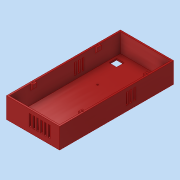
# Autodesk Inventor part: power_supply_case
Saved by Autodesk Inventor 2022 (Build 260153000, 153)
## iProperties
Created: 2020-11-03
Part Number: power_supply_case
Material: Generic
Document SubType Name: Modeling
Designer: nnico
Density: 1 g/cm^3
Appearance: Red
Author: nnico
Autodesk Inventor part; units mm, degrees
ref_plane "YZ Plane" through (0, 0, 0) normal (1, 0, 0) x (0, 1, 0)
ref_plane "XZ Plane" through (0, 0, 0) normal (0, 1, 0) x (-1, 0, 0)
ref_plane "XY Plane" through (0, 0, 0) normal (0, 0, 1) x (1, 0, 0)
sketch "Sketch1" plane through (0, 0, 0) normal (0, 1, 0) x (-1, 0, 0)
  line L0 (70, -150) -> (-70, -150)
  line L1 (-70, -150) -> (-70, 150)
  line L2 (-70, 150) -> (70, 150)
  line L3 (70, 150) -> (70, -150)
  line L4 (0, -150) -> (0, 150) construction
  line L5 (70, 0) -> (-70, 0) construction
  point P0 (0, 0)
  point P1 (0, 0)
  dimension "d0" = 140
  dimension "d1" = 300
  constraints: 12 end point, 5 midpoint, 2 parallel, 1 coincident, 1 horizontal, 1 perpendicular
  measures "d0" distance of L1.end L2.end
  measures "d1" distance of L0.end L1.end
extrude "Extrusion1" add sketch "Sketch1" along normal blind 4
sketch "Sketch2" plane through (0, 4, 0) normal (0, 1, 0) x (1, 0, 0)
  line L0 (-70, -150) -> (70, -150) projected
  line L1 (70, -150) -> (70, 150) projected
  line L2 (-70, -150) -> (70, -150)
  line L3 (70, -150) -> (70, 150)
  line L4 (70, 150) -> (-70, 150)
  line L5 (-70, 150) -> (-70, -150)
  line L6 (-66, -146) -> (66, -146)
  line L7 (66, -146) -> (66, 146)
  line L8 (66, 146) -> (-66, 146)
  line L9 (-66, 146) -> (-66, -146)
  point P0 (0, 0)
  dimension "d4" = 4
  dimension "d5" = 4
  dimension "d6" = 4
  dimension "d7" = 4
  constraints: 16 end point, 4 parallel, 2 horizontal, 2 perpendicular
  measures "d4" distance between parallel lines of L5 L9
  measures "d5" distance between parallel lines of L1 L7
  measures "d6" distance between parallel lines of L6 L0
  measures "d7" distance between parallel lines of L4 L8
extrude "Extrusion2" add sketch "Sketch2" along normal blind 50
sketch "Sketch3" plane through (0, 54, 0) normal (0, 1, 0) x (1, 0, 0)
  line L0 (-70, 150) -> (-70, -150) projected
  line L1 (-70, -90) -> (-60, -90)
  line L2 (-60, -90) -> (-60, -80)
  line L3 (-60, -80) -> (-70, -80)
  line L4 (-70, -80) -> (-70, -90)
  line L5 (-70, -150) -> (70, -150) projected
  line L6 (0, -150) -> (0, 150) construction
  line L7 (-70, 150) -> (70, 150) construction
  line L8 (70, -150) -> (70, 150) construction
  line L9 (70, 0) -> (-70, 0) construction
  line L10 (-70, 90) -> (-60, 90)
  line L11 (-60, 90) -> (-60, 80)
  line L12 (-60, 80) -> (-70, 80)
  line L13 (-70, 80) -> (-70, 90)
  line L14 (70, -90) -> (60, -90)
  line L15 (60, -90) -> (60, -80)
  line L16 (60, -80) -> (70, -80)
  line L17 (70, -80) -> (70, -90)
  line L18 (60, 90) -> (60, 80)
  line L19 (70, 90) -> (60, 90)
  line L20 (70, 80) -> (70, 90)
  line L21 (60, 80) -> (70, 80)
  line L22 (65, 80) -> (65, 90) construction
  line L23 (60, 85) -> (70, 85) construction
  circle A0 centre (65, 85) radius 2.5
  circle A1 centre (-65, 85) radius 2.5
  circle A2 centre (65, -85) radius 2.5
  circle A3 centre (-65, -85) radius 2.5
  point P0 (0, 0)
  dimension "d10" = 10
  dimension "d11" = 10
  dimension "d12" = 60
  dimension "d15" = 5
  constraints: 40 end point, 15 symmetric about line, 9 midpoint, 4 centre point, 2 parallel, 1 horizontal, 1 perpendicular, 1 point on line, 3 other
  measures "d10" distance of L3.end L2.end
  measures "d11" distance of L2.end L1.end
  measures "d12" distance from line of L5 L1.start
  measures "d15" diameter of A0
extrude "Extrusion3" add sketch "Sketch3" against normal blind 16 contours L10 L11 L12 L0 | L3 L2 L1 L0 | L14 L15 L16 L17 | L19 L20 L21 L18 | A0 | A1 | A2 | A3
sketch "Sketch4" plane through (0, 54, 0) normal (0, 1, 0) x (1, 0, 0)
  line L0 (70, -150) -> (-70, -150) construction
  line L1 (0, -150) -> (0, 150) construction
  line L2 (-70, 150) -> (70, 150) construction
  line L3 (70, -150) -> (70, 150) construction
  line L4 (70, 0) -> (-70, 0) construction
  line L5 (-70, -150) -> (-70, 150) construction
  line L6 (60, 90) -> (66, 90) construction
  line L7 (60, 90) -> (70, 90) construction
  line L8 (70, 90) -> (70, 80) construction
  line L9 (70, 80) -> (60, 80) construction
  line L10 (60, 80) -> (60, 90) construction
  line L11 (66, 80) -> (60, 80) construction
  line L12 (65, 90) -> (65, 80) construction
  line L13 (60, 80) -> (60, 90) construction
  line L14 (60, 85) -> (70, 85) construction
  circle A0 centre (65, 85) radius 2.5
  circle A1 centre (-65, 85) radius 2.5
  circle A2 centre (65, -85) radius 2.5
  circle A3 centre (-65, -85) radius 2.5
  point P0 (0, 0)
  dimension "d16" = 5
  constraints: 16 end point, 8 midpoint, 4 centre point, 3 symmetric about line, 2 parallel, 2 perpendicular, 2 point on line, 1 collinear, 1 horizontal, 3 other
  measures "d16" diameter of A0
extrude "Extrusion4" cut sketch "Sketch4" against normal blind 6
chamfer "Chamfer1" distance 6 angle 45 4 edges at (60, 38, -85) (60, 38, 85) (-60, 38, -85) (-60, 38, 85)
sketch "Sketch5" plane through (0, 4, 0) normal (0, 1, 0) x (1, 0, 0)
  line L0 (-70, 150) -> (70, 150) construction
  line L1 (0, 150) -> (0, -150) construction
  line L2 (70, -150) -> (-70, -150) construction
  line L3 (60, 110) -> (40, 110)
  line L4 (40, 110) -> (40, 130)
  line L5 (40, 130) -> (60, 130)
  line L6 (60, 130) -> (60, 110)
  line L7 (50, 110) -> (50, 130) construction
  line L8 (60, 120) -> (40, 120) construction
  line L9 (70, -150) -> (70, 150) construction
  line L10 (-60, 110) -> (-40, 110)
  line L11 (-40, 110) -> (-40, 130)
  line L12 (-40, 130) -> (-60, 130)
  line L13 (-60, 130) -> (-60, 110)
  point P0 (0, 0)
  dimension "d22" = 20
  dimension "d23" = 20
  dimension "d24" = 20
  dimension "d26" = 40
  constraints: 22 end point, 6 midpoint, 4 symmetric about line, 2 parallel, 1 horizontal, 1 perpendicular
  measures "d22" distance of L4.end L5.end
  measures "d23" distance of L3.end L4.end
  measures "d24" distance between parallel lines of L9 L7
  measures "d26" diameter of L5 L0
extrude "Extrusion5" cut sketch "Sketch5" against normal up to next
sketch "Sketch6" plane through (0, 4, 0) normal (0, 1, 0) x (1, 0, 0)
  line L0 (-57.5, 77.5) -> (57.5, 77.5) construction
  line L1 (57.5, 77.5) -> (57.5, -137.5) construction
  line L2 (57.5, -137.5) -> (-57.5, -137.5) construction
  line L3 (-57.5, -137.5) -> (-57.5, 77.5) construction
  line L4 (-70, 150) -> (70, 150) projected
  line L5 (0, 150) -> (0, -150) construction
  line L6 (-70, -150) -> (70, -150) projected
  line L7 (0, 77.5) -> (0, -137.5) construction
  line L8 (-25, 45) -> (25, 45) construction
  line L9 (25, 45) -> (25, -105) construction
  line L10 (25, -105) -> (-25, -105) construction
  line L11 (-25, -105) -> (-25, 45) construction
  line L12 (0, 45) -> (0, -105) construction
  circle A0 centre (-25, 45) radius 2.25
  circle A1 centre (25, 45) radius 2.25
  circle A2 centre (-25, -105) radius 2.25
  circle A3 centre (25, -105) radius 2.25
  line L13 (-66, -146) -> (66, -146) projected
  point P0 (0, 0)
  dimension "d29" = 115
  dimension "d30" = 215
  dimension "d31" = 50
  dimension "d32" = 150
  dimension "d33" = 32.5
  dimension "d34" = 4.5
  dimension "d35" = 4.5
  dimension "d36" = 4.5
  dimension "d37" = 4.5
  dimension "d38" = 8.5
  constraints: 22 end point, 6 midpoint, 4 centre point, 4 coincident, 4 parallel, 2 collinear, 2 horizontal, 2 perpendicular
  measures "d29" distance of L1.end L2.end
  measures "d30" distance of L0.end L1.end
  measures "d31" distance of L9.end L10.end
  measures "d32" distance of L8.end L9.end
  measures "d33" distance between parallel lines of L10 L2
  measures "d34" diameter of A0
  measures "d35" diameter of A1
  measures "d36" diameter of A2
  measures "d37" diameter of A3
  measures "d38" distance between parallel lines of L2 L13
extrude "Extrusion6" cut sketch "Sketch6" against normal up to next
sketch "Sketch7" plane through (-70, 0, 150) normal (0, 0, 1) x (1, 0, 0)
  line L0 (70, 44) -> (70, 14)
  line L1 (0, 54) -> (140, 54) projected
  line L2 (140, 0) -> (140, 54) projected
  line L3 (75, 14) -> (75, 44)
  line L4 (80, 14) -> (80, 44)
  line L5 (85, 14) -> (85, 44)
  line L6 (90, 14) -> (90, 44)
  line L7 (95, 14) -> (95, 44)
  line L8 (100, 14) -> (100, 44)
  line L9 (105, 14) -> (105, 44)
  line L10 (110, 14) -> (110, 44)
  line L11 (115, 14) -> (115, 44)
  line L12 (75, 44) -> (70, 44)
  line L13 (85, 44) -> (80, 44)
  line L14 (95, 44) -> (90, 44)
  line L15 (115, 44) -> (110, 44)
  line L16 (105, 44) -> (100, 44)
  line L17 (70, 14) -> (75, 14)
  line L18 (80, 14) -> (85, 14)
  line L19 (90, 14) -> (95, 14)
  line L20 (100, 14) -> (105, 14)
  line L21 (110, 14) -> (115, 14)
  line L22 (60, 44) -> (60, 14)
  line L23 (65, 14) -> (65, 44)
  line L24 (65, 44) -> (60, 44)
  line L25 (60, 14) -> (65, 14)
  point P0 (70, 0)
  dimension "d42" = 30
  dimension "d45" = 5
  dimension "d47" = 5
  dimension "d48" = 5
  dimension "d49" = 5
  dimension "d50" = 5
  dimension "d51" = 5
  dimension "d52" = 5
  dimension "d53" = 5
  dimension "d54" = 10
  dimension "d55" = 25
  dimension "d56" = 5
  dimension "d60" = 30
  dimension "d61" = 5
  dimension "d62" = 5
  constraints: 48 end point, 13 collinear, 12 perpendicular, 8 horizontal
  measures "d42" distance of L0.end L0.start
  measures "d45" distance of L3.end L0.start
  measures "d47" distance of L11.end L10.end
  measures "d48" distance of L9.end L10.end
  measures "d49" distance of L8.end L9.end
  measures "d50" distance of L7.end L8.end
  measures "d51" distance of L6.end L7.end
  measures "d52" distance of L5.end L6.end
  measures "d53" distance of L4.end L5.end
  measures "d54" distance from line of L1 L11.end
  measures "d55" horizontal distance of L1.end L11.end
  measures "d56" distance of L3.end L4.end
  measures "d60" distance of L22.end L24.end
  measures "d61" distance of L24.start L24.end
  measures "d62" distance of L0.start L24.start
extrude "Extrusion7" cut sketch "Sketch7" against normal up to next
sketch "Sketch9" plane through (70, 0, 150) normal (1, 0, 0) x (0, 0, -1)
  line L0 (175, 44) -> (180, 44)
  line L1 (180, 44) -> (180, 14)
  line L2 (180, 14) -> (175, 14)
  line L3 (175, 14) -> (175, 44)
  line L4 (0, 54) -> (300, 54) projected
  line L5 (185, 44) -> (190, 44)
  line L6 (190, 44) -> (190, 14)
  line L7 (190, 14) -> (185, 14)
  line L8 (185, 14) -> (185, 44)
  line L9 (195, 44) -> (200, 44)
  line L10 (200, 44) -> (200, 14)
  line L11 (200, 14) -> (195, 14)
  line L12 (195, 14) -> (195, 44)
  line L13 (300, 0) -> (300, 54) projected
  point P0 (150, 0)
  dimension "d63" = 5
  dimension "d64" = 30
  dimension "d65" = 10
  dimension "d68" = 5
  dimension "d69" = 30
  dimension "d70" = 5
  dimension "d71" = 30
  dimension "d72" = 5
  dimension "d73" = 5
  dimension "d74" = 100
  constraints: 24 end point, 6 parallel, 3 horizontal, 3 perpendicular, 2 collinear
  measures "d63" distance of L1.end L2.end
  measures "d64" distance of L0.end L1.end
  measures "d65" distance from line of L4 L0.start
  measures "d68" distance of L6.end L8.start
  measures "d69" distance of L5.end L6.end
  measures "d70" distance of L10.end L12.start
  measures "d71" distance of L9.end L10.end
  measures "d72" distance of L8.end L0.end
  measures "d73" distance of L12.end L5.end
  measures "d74" distance from line of L13 L9.end
extrude "Extrusion8" cut sketch "Sketch9" against normal blind 140
body "Solid1"
